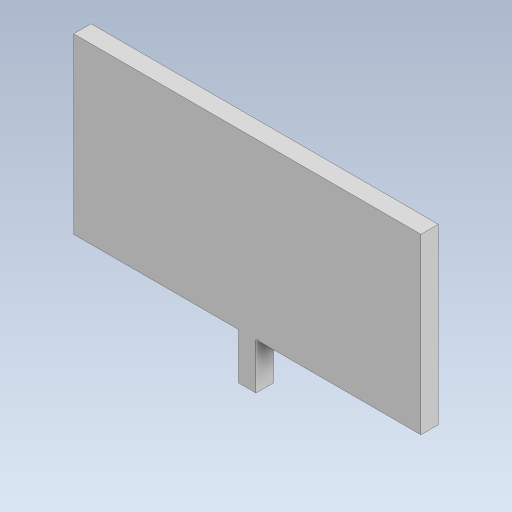
# Autodesk Inventor part: 零件11
Saved by Autodesk Inventor 2023 (Build 270158000, 158)
## iProperties
Created: 2023-05-16
Part Number: 零件11
Material: 一般
Document SubType Name: Modeling
Designer: Johnny Jou
Density: 1 g/cm^3
Appearance: 預設
Author: Johnny Jou
Autodesk Inventor part; units mm, degrees
ref_plane "YZ Plane" through (0, 0, 0) normal (1, 0, 0) x (0, 1, 0)
ref_plane "XZ Plane" through (0, 0, 0) normal (0, 1, 0) x (-1, 0, 0)
ref_plane "XY Plane" through (0, 0, 0) normal (0, 0, 1) x (1, 0, 0)
sketch "草圖1" plane through (0, 0, 0) normal (0, 0, 1) x (1, 0, 0)
  line L0 (0, 0) -> (60, 0)
  line L1 (60, 0) -> (60, 30)
  line L2 (60, 30) -> (0, 30)
  line L3 (0, 30) -> (0, 0)
  line L4 (28.5, 0) -> (31.5, 0)
  line L5 (31.5, 0) -> (31.5, -8)
  line L6 (31.5, -8) -> (28.5, -8)
  line L7 (28.5, -8) -> (28.5, 0)
  point P0 (30, -8)
  point P1 (30, 0)
  dimension "d0" = 60
  dimension "d1" = 30
  dimension "d2" = 3
  dimension "d3" = 8
  constraints: 16 end point, 4 parallel, 2 horizontal, 2 midpoint, 2 perpendicular, 1 point on line, 1 vertical alignment
  measures "d0" distance of L1.end L2.end
  measures "d1" distance of L0.end L1.end
  measures "d2" distance between parallel lines of L7 L5
  measures "d3" distance of L4.end L5.end
extrude "擠出1" add sketch "草圖1" along normal blind 3
